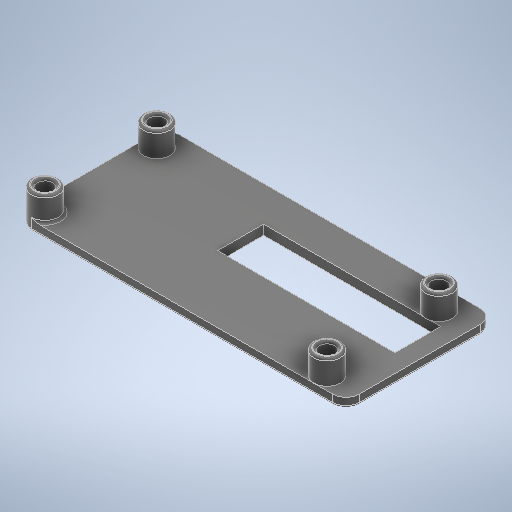
# Autodesk Inventor part: PiMountBracket
Saved by Autodesk Inventor 2025 (Build 290162000, 162)
## iProperties
Created: 2025-02-27
Part Number: PiMountBracket
Material: ABS Plastic
Document SubType Name: Modeling
Designer: tvoko
Density: 1.06 g/cm^3
Appearance: Smooth - Black
Author: tvoko
Autodesk Inventor part; units mm, degrees
ref_plane "YZ Plane" through (0, 0, 0) normal (1, 0, 0) x (0, 1, 0)
ref_plane "XZ Plane" through (0, 0, 0) normal (0, 1, 0) x (-1, 0, 0)
ref_plane "XY Plane" through (0, 0, 0) normal (0, 0, 1) x (1, 0, 0)
sketch "Sketch1" plane through (0, 0, 0) normal (0, 1, 0) x (-1, 0, 0)
  line L0 (0, 0) -> (-58, 0) construction
  line L1 (-58, 0) -> (-58, -23) construction
  line L2 (-58, -23) -> (0, -23) construction
  line L3 (0, -23) -> (0, 0) construction
  circle A0 centre (0, -23) radius 1.6
  circle A1 centre (-58, -23) radius 1.6
  circle A2 centre (-58, 0) radius 1.6
  circle A3 centre (0, 0) radius 1.6
  circle A4 centre (0, -23) radius 2.75
  circle A5 centre (-58, -23) radius 2.75
  circle A6 centre (-58, 0) radius 2.75
  circle A7 centre (0, 0) radius 2.75
  line L4 (2.75, -23) -> (2.75, 0)
  line L5 (0, 2.75) -> (-58, 2.75)
  line L6 (-60.75, 0) -> (-60.75, -23) construction
  line L7 (-58, -25.75) -> (0, -25.75) construction
  line L8 (-24.55, -20.4) -> (-60.95, -20.4)
  line L9 (-60.95, -20.4) -> (-60.95, -11)
  line L10 (-60.95, -11) -> (-24.55, -11)
  line L11 (-24.55, -11) -> (-24.55, -20.4)
  line L12 (2.75, -23) -> (2.75, -24.9)
  line L13 (0, -27.65) -> (-61.9, -27.65)
  line L14 (-64.65, -24.9) -> (-64.65, 0)
  line L15 (-61.9, 2.75) -> (-58, 2.75)
  arc A8 (0, -27.65) -> (2.75, -24.9) centre (0, -24.9) ccw
  arc A9 (-64.65, -24.9) -> (-61.9, -27.65) centre (-61.9, -24.9) ccw
  arc A10 (-61.9, 2.75) -> (-64.65, 0) centre (-61.9, 0) ccw
  line L16 (-24.55, -15.7) -> (-60.95, -15.7) construction
  point P0 (-57.1042, -20.4)
  point P1 (-58.8958, -20.4)
  dimension "d0" = 3.2
  dimension "d1" = 58
  dimension "d2" = 23
  dimension "d3" = 5.5
  dimension "d12" = 36.4
  dimension "d13" = 9.4
  dimension "d15" = 2.75
  dimension "d16" = 4.65
  dimension "d17" = 6.65
  dimension "d18" = 11.95
  dimension "d19" = 0.2
  constraints: 34 end point, 15 tangent, 14 point on circle, 11 centre point, 9 equal radius, 8 coincident, 5 perpendicular, 4 parallel, 3 horizontal, 2 midpoint, 1 vertical
  measures "d0" diameter of A0
  measures "d1" distance of L1.end L2.end
  measures "d2" distance of L2.end L0.start
  measures "d3" diameter of A4
  measures "d12" distance of L8.start L8.end
  measures "d13" distance of L8.end L9.end
  measures "d15" radius of A8
  measures "d16" distance between parallel lines of L13 L2
  measures "d17" distance between parallel lines of L14 L1
  measures "d18" distance between parallel lines of L16 L13
  measures "d19" distance between parallel lines of L6 L9
extrude "Extrusion1" add sketch "Sketch1" against normal blind 2 contours A4 | A6 | L12 A8 L13 A9 L14 A10 L15 L5 A7 L4 | A7 | A5 L8 picked at (-58.0643, -20.7372)
extrude "Extrusion2" add sketch "Sketch1" along normal blind 5 contours A4 | A6 | A7 | A5 L8 | L8 A5
fillet "Fillet1" radius 0.5 14 edges at (1.9445, 0, -1.9445) (60.75, 5, -23) (60.75, 5, 0) (2.75, 5, -23) (1.6, 5, -23) (1.6, 5, 0) (2.75, 5, 0) (59.6, 5, -23) (59.6, 5, 0) (-1.9445, -2, 1.9445) (1.6, -2, -23) (1.6, -2, 0) (59.6, -2, 0) (59.6, -2, -23)
body "Solid1"
